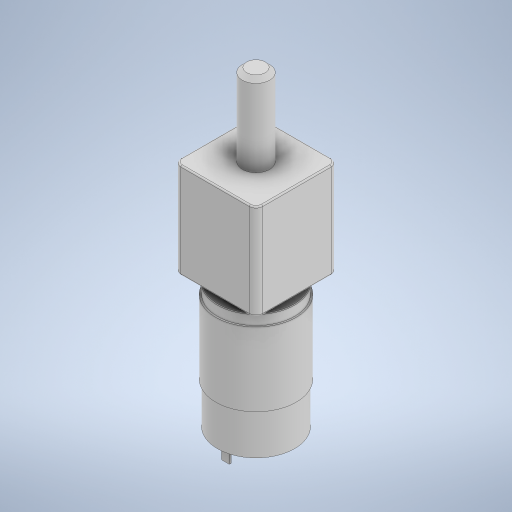
# Autodesk Inventor part: DC Motor
Saved by Autodesk Inventor 2024 (Build 280153000, 153)
## iProperties
Created: 2023-10-10
Part Number: DC Motor
Material: Generic
Document SubType Name: Modeling
Designer: luke.macenski3281
Density: 1 g/cm^3
Appearance: Default
Author: luke.macenski3281
Autodesk Inventor part; units mm, degrees
ref_plane "YZ Plane" through (0, 0, 0) normal (1, 0, 0) x (0, 1, 0)
ref_plane "XZ Plane" through (0, 0, 0) normal (0, 1, 0) x (-1, 0, 0)
ref_plane "XY Plane" through (0, 0, 0) normal (0, 0, 1) x (1, 0, 0)
sketch "Sketch1" plane through (0, 0, 0) normal (0, 1, 0) x (-1, 0, 0)
  circle A0 centre (0, 0) radius 17.9705
  dimension "d0" = 35.941
  constraints: 1 centre point, 1 coincident
  measures "d0" diameter of A0
extrude "Extrusion1" add sketch "Sketch1" along normal blind 19.177
sketch "Sketch2" plane through (0, 19.177, 0) normal (0, 1, 0) x (1, 0, 0)
  circle A0 centre (0, 0) radius 18.7325
  dimension "d3" = 37.465
  constraints: 1 centre point, 1 coincident
  measures "d3" diameter of A0
extrude "Extrusion2" add sketch "Sketch2" along normal blind 34.29
sketch "Sketch3" plane through (0, 53.467, 0) normal (0, 1, 0) x (1, 0, 0)
  circle A0 centre (0, 0) radius 17.9705
  dimension "d6" = 35.941
  constraints: 1 centre point, 1 coincident
  measures "d6" diameter of A0
extrude "Extrusion3" add sketch "Sketch3" along normal blind 4.826
sketch "Sketch4" plane through (0, 58.293, 0) normal (0, 1, 0) x (1, 0, 0)
  circle A0 centre (0, 0) radius 6.477
  dimension "d9" = 12.954
  constraints: 1 centre point, 1 coincident
  measures "d9" diameter of A0
extrude "Extrusion4" add sketch "Sketch4" along normal blind 4.318
sketch "Sketch5" plane through (0, 62.611, 0) normal (0, 1, 0) x (1, 0, 0)
  circle A0 centre (0, 0) radius 1.5875
  dimension "d12" = 3.175
  constraints: 1 centre point, 1 coincident
  measures "d12" diameter of A0
extrude "Extrusion5" add sketch "Sketch5" along normal blind 8.2804
fillet "Fillet1" radius 0.3175 1 edges at (-17.9705, 58.293, 0)
fillet "Fillet2" radius 0.3175 1 edges at (-1.5875, 70.8914, 0)
sketch "Sketch6" plane through (0, 0, 0) normal (0, -1, 0) x (1, 0, 0)
  circle A0 centre (0, 0) radius 1.5875 projected
  circle A1 centre (0, 0) radius 6.5024
  dimension "d17" = 13.0048
  constraints: 1 centre point, 1 coincident
  measures "d17" diameter of A1
extrude "Extrusion6" add sketch "Sketch6" along normal blind 3.6576 contours A0 | A1
sketch "Sketch7" plane through (0, -3.6576, 0) normal (0, -1, 0) x (1, 0, 0)
  circle A0 centre (0, 0) radius 1.5875 projected
  circle A1 centre (0, 0) radius 1.5875
  constraints: 1 centre point, 1 coincident
extrude "Extrusion7" add sketch "Sketch7" along normal blind 1.8542
fillet "Fillet3" radius 0.635 2 edges at (-6.5024, -3.6576, 0) (-1.5875, -5.5118, 0)
sketch "Sketch8" plane through (0, 0, 0) normal (0, -1, 0) x (1, 0, 0)
  line L0 (1.9177, 13.5128) -> (-1.9177, 13.5128)
  line L1 (-1.9177, 13.5128) -> (-1.9177, 14.1478)
  line L2 (-1.9177, 14.1478) -> (1.9177, 14.1478)
  line L3 (1.9177, 14.1478) -> (1.9177, 13.5128)
  line L4 (1.9177, 13.5128) -> (-1.9177, 14.1478) construction
  line L5 (-1.9177, 13.5128) -> (1.9177, 14.1478) construction
  line L6 (1.9177, -14.1478) -> (-1.9177, -14.1478)
  line L7 (-1.9177, -14.1478) -> (-1.9177, -13.5128)
  line L8 (-1.9177, -13.5128) -> (1.9177, -13.5128)
  line L9 (1.9177, -13.5128) -> (1.9177, -14.1478)
  line L10 (1.9177, -14.1478) -> (-1.9177, -13.5128) construction
  line L11 (-1.9177, -14.1478) -> (1.9177, -13.5128) construction
  circle A0 centre (0, 0) radius 6.5024 projected
  circle A1 centre (0, 0) radius 0.9525 projected
  line L12 (0, 0) -> (0, -10.7533)
  point P0 (0, 13.8303)
  point P1 (0, -13.8303)
  point P2 (0, -14.1478)
  point P3 (0, 14.1478)
  point P4 (-1.9177, -13.8303)
  point P5 (1.9177, -13.8303)
  point P6 (-1.9177, 13.8303)
  point P7 (1.9177, 13.8303)
  point P8 (0, -13.5128)
  dimension "d24" = 13.5128
  dimension "d26" = 0.635
  dimension "d27" = 0.635
  dimension "d28" = 13.5128
  dimension "d29" = 3.8354
  dimension "d30" = 3.8354
  dimension "d31" = 0
  constraints: 26 end point, 11 midpoint, 4 parallel, 2 horizontal, 2 perpendicular, 1 point on line, 1 vertical
  measures "d24" distance from line of L8 A0.centre
  measures "d26" distance between parallel lines of L2 L0
  measures "d27" distance between parallel lines of L8 L6
  measures "d28" distance from line of L12.start L0
  measures "d29" distance of point (-1.918, -13.83) point (1.918, -13.83)
  measures "d30" distance of point (-1.918, 13.83) point (1.918, 13.83)
  measures "d31" distance from line of L12 point (0, -13.513)
extrude "Extrusion8" add sketch "Sketch8" along normal blind 7.366 contours L0 L1 L2 L3 | L6 L7 L8 L9
fillet "Fillet4" radius 0.3175 4 edges at (1.9177, -7.366, 13.8303) (-1.9177, -7.366, 13.8303) (1.9177, -7.366, -13.8303) (-1.9177, -7.366, -13.8303)
sketch "Sketch9" plane through (0, 62.611, 0) normal (0, 1, 0) x (1, 0, 0)
  line L0 (-19.1135, 19.1135) -> (19.1135, 19.1135)
  line L1 (19.1135, 19.1135) -> (19.1135, -19.1135)
  line L2 (19.1135, -19.1135) -> (-19.1135, -19.1135)
  line L3 (-19.1135, -19.1135) -> (-19.1135, 19.1135)
  circle A0 centre (0, 0) radius 1.5875 projected
  line L4 (-19.1135, 19.1135) -> (19.1135, -19.1135) construction
  line L5 (19.1135, 19.1135) -> (-19.1135, -19.1135) construction
  dimension "d35" = 38.227
  dimension "d36" = 38.227
  constraints: 12 end point, 2 midpoint, 2 parallel, 1 horizontal, 1 perpendicular
  measures "d35" distance of L2.end L0.start
  measures "d36" distance between parallel lines of L1 L3
extrude "Extrusion9" add sketch "Sketch9" along normal blind 44.45
fillet "Fillet5" radius 3.175 4 edges at (19.1135, 84.836, 19.1135) (-19.1135, 84.836, 19.1135) (19.1135, 84.836, -19.1135) (-19.1135, 84.836, -19.1135)
fillet "Fillet6" radius 0.635 16 edges at (-18.1836, 62.611, 18.1836) (0, 62.611, 19.1135) (18.1836, 62.611, 18.1836) (19.1135, 62.611, 0) (18.1836, 62.611, -18.1836) (0, 62.611, -19.1135) (-18.1836, 62.611, -18.1836) (-19.1135, 62.611, 0) (-18.1836, 107.061, 18.1836) (0, 107.061, 19.1135) (18.1836, 107.061, 18.1836) (19.1135, 107.061, 0) (18.1836, 107.061, -18.1836) (0, 107.061, -19.1135) (-18.1836, 107.061, -18.1836) (-19.1135, 107.061, 0)
sketch "Sketch10" plane through (0, 107.061, 0) normal (0, 1, 0) x (1, 0, 0)
  circle A0 centre (0, 0) radius 1.5875 projected
  circle A1 centre (0, 0) radius 6.35
  line L0 (-0.892, -6.8107) -> (1.3528, -6.8107)
  line L1 (1.3528, -6.8107) -> (1.3528, -5.4272)
  line L2 (1.3528, -5.4272) -> (-0.892, -5.4272)
  line L3 (-0.892, -5.4272) -> (-0.892, -6.8107)
  dimension "d41" = 12.7
  constraints: 8 end point, 2 parallel, 1 centre point, 1 coincident, 1 horizontal, 1 perpendicular
  measures "d41" diameter of A1
extrude "Extrusion10" add sketch "Sketch10" along normal blind 38.1 contours A0 | A1 L1 L2 L3 | L3 L2 L1 A1
chamfer "Chamfer1" distance 2.032 angle 45 1 edges at (-6.35, 145.161, 0)
body "Solid1"
